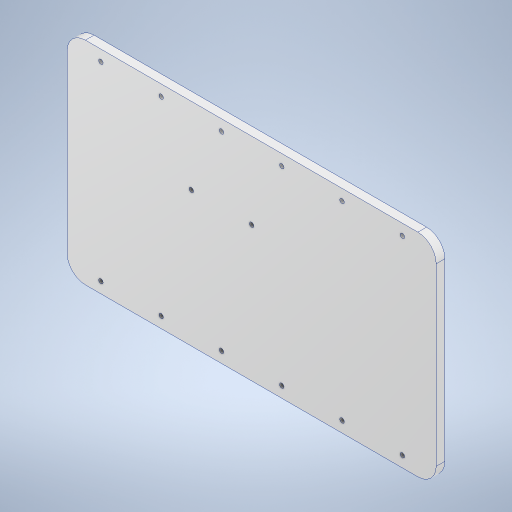
# Autodesk Inventor part: Class-D RevA Board Heatsink
Saved by Autodesk Inventor 2024 (Build 280153000, 153)
## iProperties
Created: 2023-08-05
Part Number: Class-D RevA Board Heatsink
Material: Aluminum 6061
Document SubType Name: Modeling
Designer: Ishaan
Density: 2.7 g/cm^3
Appearance: Aluminum - Flat
Author: Ishaan
Autodesk Inventor part; units mm, degrees
ref_plane "YZ Plane" through (0, 0, 0) normal (1, 0, 0) x (0, 1, 0)
ref_plane "XZ Plane" through (0, 0, 0) normal (0, 1, 0) x (-1, 0, 0)
ref_plane "XY Plane" through (0, 0, 0) normal (0, 0, 1) x (1, 0, 0)
sketch "Sketch1" plane through (0, 0, 0) normal (0, 0, 1) x (1, 0, 0)
  line L0 (-99, -56) -> (99, -56)
  line L1 (99, -56) -> (99, 56)
  line L2 (99, 56) -> (-99, 56)
  line L3 (-99, 56) -> (-99, -56)
  line L4 (-99, -56) -> (99, 56) construction
  line L5 (99, -56) -> (-99, 56) construction
  line L6 (-99, -56) -> (8.25, -56)
  line L7 (8.25, -56) -> (8.25, 20)
  line L8 (8.25, 20) -> (-99, 20)
  line L9 (-99, 20) -> (-99, -56)
  line L10 (8.25, 20) -> (8.25, 56)
  point P0 (0, 0)
  dimension "d0" = 112
  dimension "d1" = 198
  dimension "d3" = 76
  dimension "d50" = 8.25
  constraints: 22 end point, 4 parallel, 3 perpendicular, 2 horizontal, 2 midpoint, 1 point on line
  measures "d0" distance of L0.end L1.end
  measures "d1" distance of L1.end L2.end
  measures "d3" distance of L6.end L7.end
  measures "d50" distance from line of L10 point (0, 0)
extrude "Extrusion1" add sketch "Sketch1" along normal blind 4.7625
sketch "Sketch2" plane through (0, 0, 4.7625) normal (0, 0, 1) x (1, 0, 0)
  line L0 (-99, -56) -> (99, -56) projected
  line L1 (-99, 56) -> (-99, -56) projected
  line L2 (99, 56) -> (-99, 56) projected
  line L3 (99, -56) -> (99, 56) projected
  line L4 (-16.5, -52) -> (16.5, -52) construction
  line L5 (-49.5, -52) -> (-16.5, -52) construction
  line L6 (8.25, 20) -> (-99, 20) projected
  point P0 (0, 0)
  point P1 (-82.5, -52)
  point P2 (49.5, -52)
  point P3 (-82.5, 52)
  point P4 (-49.5, 52)
  point P5 (-16.5, 52)
  point P6 (16.5, 52)
  point P7 (49.5, 52)
  point P8 (82.5, -52)
  point P9 (82.5, 52)
  point P10 (-33, 16)
  point P11 (0, 16)
  point P12 (0, -52)
  point P13 (-33, -52)
  dimension "d6" = 4
  dimension "d9" = 33
  dimension "d12" = 104
  dimension "d15" = 4
  dimension "d17" = 16.5
  dimension "d18" = 16.5
  dimension "d51" = 4
  constraints: 4 end point, 3 horizontal, 2 midpoint, 2 vertical alignment, 1 coincident, 1 horizontal alignment, 1 vertical, 11 other
  measures "d6" distance from line of point (-82.5, -52) L0
  measures "d9" distance of point (-82.5, -52) L5.start
  measures "d12" distance of point (-82.5, -52) point (-82.5, 52)
  measures "d15" distance from line of L2 point (-82.5, 52)
  measures "d17" distance from line of point (-82.5, -52) L1
  measures "d18" distance from line of point (82.5, -52) L3
  measures "d51" distance from line of L6 point (-33, 16)
hole "Hole1" at (-82.5, -52, 4.7625) at (-49.5, -52, 4.7625) at (-16.5, -52, 4.7625) at (16.5, -52, 4.7625) at (49.5, -52, 4.7625) at (-82.5, 52, 4.7625) at (-49.5, 52, 4.7625) at (-16.5, 52, 4.7625) at (16.5, 52, 4.7625) at (49.5, 52, 4.7625) at (82.5, -52, 4.7625) at (82.5, 52, 4.7625) at (-33, 16, 4.7625) at (0, 16, 4.7625) direction (0, 0, -1) diameter 2.459 end through all thread size "M3x0.5" class "6H" standard "ANSI Metric M Profile"
fillet "Fillet4" radius 8 4 edges at (99, -56, 2.3813) (-99, -56, 2.3813) (-99, 56, 2.3813) (99, 56, 2.3813)
sketch "Sketch6" plane through (0, 0, 4.7625) normal (0, 0, 1) x (1, 0, 0)
  arc A0 (99, 48) -> (91, 56) centre (91, 48) ccw projected
  line L0 (91, 56) -> (-91, 56) projected
  arc A1 (-91, 56) -> (-99, 48) centre (-91, 48) ccw projected
  line L1 (-99, 48) -> (-99, -48) projected
  arc A2 (-99, -48) -> (-91, -56) centre (-91, -48) ccw projected
  line L2 (-91, -56) -> (91, -56) projected
  arc A3 (91, -56) -> (99, -48) centre (91, -48) ccw projected
  line L3 (99, -48) -> (99, 48) projected
  circle A4 centre (0, 16) radius 1.2295 projected
  circle A5 centre (-33, 16) radius 1.2295 projected
  circle A6 centre (82.5, 52) radius 1.2295 projected
  circle A7 centre (82.5, -52) radius 1.2295 projected
  circle A8 centre (49.5, 52) radius 1.2295 projected
  circle A9 centre (16.5, 52) radius 1.2295 projected
  circle A10 centre (-16.5, 52) radius 1.2295 projected
  circle A11 centre (-49.5, 52) radius 1.2295 projected
  circle A12 centre (-82.5, 52) radius 1.2295 projected
  circle A13 centre (49.5, -52) radius 1.2295 projected
  circle A14 centre (16.5, -52) radius 1.2295 projected
  circle A15 centre (-16.5, -52) radius 1.2295 projected
  circle A16 centre (-49.5, -52) radius 1.2295 projected
  circle A17 centre (-82.5, -52) radius 1.2295 projected
  line L4 (-91, 58) -> (91, 58)
  arc A18 (101, 48) -> (91, 58) centre (91, 48) ccw
  line L5 (101, 48) -> (101, -48)
  arc A19 (91, -58) -> (101, -48) centre (91, -48) ccw
  line L6 (91, -58) -> (-91, -58)
  arc A20 (-101, -48) -> (-91, -58) centre (-91, -48) ccw
  line L7 (-101, -48) -> (-101, 48)
  arc A21 (-91, 58) -> (-101, 48) centre (-91, 48) ccw
  point P0 (0, 0)
  dimension "d53" = 2
  constraints: 8 end point, 8 point on circle, 4 centre point, 7 other
  measures "d53" distance between parallel lines of L0 L4
extrude "Extrusion3" add sketch "Sketch6" against normal up to surface (4.7625 mm away) contours L4 A18 L5 A19 L6 A20 L7 A21
sketch "Sketch3" plane through (0, 0, 4.7625) normal (0, 0, 1) x (1, 0, 0)
  circle A0 centre (0, 16) radius 1.7 projected
  circle A1 centre (-33, 16) radius 1.7 projected
  circle A2 centre (82.5, 52) radius 1.7 projected
  circle A3 centre (82.5, -52) radius 1.7 projected
  circle A4 centre (49.5, 52) radius 1.7 projected
  circle A5 centre (16.5, 52) radius 1.7 projected
  circle A6 centre (49.5, -52) radius 1.7 projected
  circle A7 centre (16.5, -52) radius 1.7 projected
  circle A8 centre (-16.5, -52) radius 1.7 projected
  circle A9 centre (-49.5, -52) radius 1.7 projected
  circle A10 centre (-82.5, -52) radius 1.7 projected
  line L0 (99, 56) -> (-99, 56) projected
  line L1 (-99, 56) -> (-99, -56) projected
  line L2 (-99, -56) -> (99, -56) projected
  line L3 (99, -56) -> (99, 56) projected
  line L4 (99, 23) -> (0, 23) construction
  line L5 (99, 10) -> (-99, 10) construction
  line L6 (90.5, -56) -> (90.5, 10)
  line L7 (99, 23) -> (80.5, 23)
  line L8 (80.5, 23) -> (80.5, 10)
  line L9 (90.5, 10) -> (80.5, 10)
  line L10 (63.5, 10) -> (80.5, 10)
  line L11 (80.5, 10) -> (80.5, 23)
  line L12 (80.5, 23) -> (63.5, 23)
  line L13 (63.5, 23) -> (63.5, 10)
  line L14 (63.5, 10) -> (80.5, 23) construction
  line L15 (80.5, 10) -> (63.5, 23) construction
  point P0 (0, 0)
  point P1 (82.5, 27)
  point P2 (72, 16.5)
  dimension "d29" = 4
  dimension "d30" = 8
  dimension "d31" = 4
  dimension "d32" = 4
  dimension "d33" = 2
  dimension "d36" = 72.5
  dimension "d37" = 17
  dimension "d38" = 13
  constraints: 24 end point, 8 point on line, 3 perpendicular, 2 collinear, 2 midpoint, 2 parallel, 2 vertical, 1 horizontal, 1 vertical alignment
  measures "d29" distance from line of L2 A3.centre
  measures "d30" distance from line of L6 A3.centre
  measures "d31" distance from line of L4 point (82.5, 27)
  measures "d32" distance from line of L0 A2.centre
  measures "d33" distance from line of L8 point (82.5, 27)
  measures "d36" distance from line of L2 point (72, 16.5)
  measures "d37" distance between parallel lines of L8 L13
  measures "d38" distance between parallel lines of L12 L10
equation "\"d15\" = d6"
equation "\"d18\" = d17"
equation "\"d31\" = d32"
body "Solid1"
